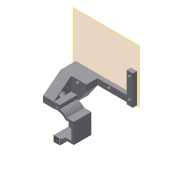
# Autodesk Inventor part: cellSTORM_v5_focusmotormount
Saved by Autodesk Inventor 2019 (Build 230136000, 136)
## iProperties
Created: 2020-05-04
Part Number: cellSTORM_v5_focusmotormount
Material: Generic
Document SubType Name: Modeling
Designer: diederichbenedict
Density: 1 g/cm^3
Appearance: Default
Author: diederichbenedict
Autodesk Inventor part; units mm, degrees
ref_plane "YZ Plane" through (0, 0, 0) normal (1, 0, 0) x (0, 1, 0)
ref_plane "XZ Plane" through (0, 0, 0) normal (0, 1, 0) x (-1, 0, 0)
ref_plane "XY Plane" through (0, 0, 0) normal (0, 0, 1) x (1, 0, 0)
ref_plane "Work Plane1" through (0, 0, 0) normal (0, 0, 1) x (1, 0, 0)
sketch "Sketch1" plane through (0, 0, 0) normal (0, 0, 1) x (1, 0, 0)
  line L0 (-45, 22) -> (22, 22) projected
  line L1 (22, 22) -> (22, -22) projected
  line L2 (22, -22) -> (-45, -22) projected
  line L3 (-45, -28) -> (-45, -22) projected
  line L4 (-30, -28) -> (-45, -28) projected
  line L5 (-30, -28) -> (-28, -30) projected
  line L6 (-28, -30) -> (28, -30) projected
  line L7 (28, -30) -> (30, -28) projected
  line L8 (30, -28) -> (30, 28) projected
  line L9 (30, 28) -> (28, 30) projected
  line L10 (28, 30) -> (-28, 30) projected
  line L11 (-28, 30) -> (-30, 28) projected
  line L12 (-30, 28) -> (-45, 28) projected
  line L13 (-45, 22) -> (-45, 28) projected
  circle A0 centre (25, 25) radius 1.95 projected
  circle A1 centre (25, 0) radius 1.95 projected
  circle A2 centre (0, 25) radius 1.95 projected
  circle A3 centre (-25, -25) radius 1.95 projected
  circle A4 centre (25, -25) radius 1.95 projected
  circle A5 centre (-25, 25) radius 1.95 projected
  circle A6 centre (0, -25) radius 1.95 projected
  line L14 (30, 4.1832) -> (22.5, 4.1832)
  line L15 (22.5, 4.1832) -> (22.5, -32.3594)
  line L16 (22.5, -32.3594) -> (30, -32.3594)
  line L17 (30, -32.3594) -> (30, 4.1832)
  line L18 (22.5, -22.5) -> (-45, -22.5)
  line L19 (-45, -22.5) -> (-45, -30)
  line L20 (-45, -30) -> (22.5, -30)
  line L21 (22.5, -30) -> (22.5, -22.5)
  circle A7 centre (25, 0) radius 2.15
  circle A8 centre (25, -25) radius 2.15
  circle A9 centre (0, -25) radius 2.15
  circle A10 centre (-25, -25) radius 2.15
  point P0 (0, 0)
  dimension "d0" = 0
  dimension "d1" = 0.5
  dimension "d2" = 0.5
  dimension "d3" = 0.2
  dimension "d4" = 0.2
  dimension "d5" = 0.2
  dimension "d6" = 0.2
  constraints: 16 end point, 4 centre point, 4 parallel, 3 point on line, 2 horizontal, 2 perpendicular
  measures "d0" distance between parallel lines of L8 L17
  measures "d1" distance between parallel lines of L1 L15
  measures "d2" distance between parallel lines of L2 L18
  measures "d3" radial gap between concentric circles of A1 A7
  measures "d4" radial gap between concentric circles of A4 A8
  measures "d5" radial gap between concentric circles of A6 A9
  measures "d6" radial gap between concentric circles of A3 A10
extrude "Extrusion1" add sketch "Sketch1" along normal blind 5 contours L18 L15 L6 L5 L4 L3 | L4 L5 L20 L19 | L15 L14 L8 L7 L6 | L6 L7 L17 L16 L15
ref_plane "Work Plane2" through (-32, -78.0277, 40.0715) normal (0, 0, -1) x (0, 1, 0)
sketch "Sketch2" plane through (-32, -78.0277, 40.0715) normal (0, 0, -1) x (0, 1, 0)
  arc A0 (1.8777, 3.5) -> (-2.3223, 3.5) centre (-0.2223, 3.5) ccw projected
  arc A1 (8.5277, 14.4287) -> (3.7223, 7) centre (17.2777, 3.5) ccw projected
  arc A2 (30.8332, 7) -> (26.0277, 14.4287) centre (17.2777, 3.5) ccw projected
  arc A3 (32.6777, 3.5) -> (36.8777, 3.5) centre (34.7777, 3.5) ccw projected
  line L0 (3.7223, 0) -> (-0.2223, 0) projected
  arc A4 (3.2777, 3.5) -> (31.2777, 3.5) centre (17.2777, 3.5) ccw projected
  line L1 (3.2065, 0) -> (-4.2223, 0)
  line L2 (-4.2223, 0) -> (-4.2223, 7.3838)
  line L3 (-4.2223, 7.3838) -> (0.0956, 7.3838)
  line L4 (31.3467, -0.0091) -> (37.7777, -0.0091)
  line L5 (37.7777, -0.0091) -> (38.7777, -0.0091)
  line L6 (38.7777, -0.0091) -> (38.7777, 7.3934)
  line L7 (38.7777, 7.3934) -> (34.4577, 7.3934)
  circle A5 centre (34.7777, 3.5) radius 1.4
  circle A6 centre (-0.2223, 3.5) radius 1.4
  line L8 (8.5277, 22) -> (8.5277, 14.4287)
  line L9 (26.0277, 22) -> (26.0277, 14.4287)
  line L10 (8.0277, 14.6664) -> (5.0277, 14.6664)
  line L11 (5.0277, 14.6664) -> (5.0277, 24.6664)
  line L12 (5.0277, 24.6664) -> (8.0277, 24.6664)
  line L13 (8.0277, 24.6664) -> (8.0277, 14.6664)
  line L14 (26.5277, 14.6664) -> (29.5277, 14.6664)
  line L15 (29.5277, 14.6664) -> (29.5277, 24.6664)
  line L16 (29.5277, 24.6664) -> (26.5277, 24.6664)
  line L17 (26.5277, 24.6664) -> (26.5277, 14.6664)
  line L18 (26.5277, 24.6664) -> (8.0277, 24.6664)
  line L19 (8.0277, 24.6664) -> (8.0277, 21.6664)
  line L20 (8.0277, 21.6664) -> (26.5277, 21.6664)
  line L21 (26.5277, 21.6664) -> (26.5277, 24.6664)
  arc A7 (31.3467, -0.0091) -> (26.5277, 14.6664) centre (17.2777, 3.5) ccw
  arc A8 (8.0277, 14.6664) -> (3.2065, 0) centre (17.2777, 3.5) ccw
  arc A9 (34.4577, 7.3934) -> (29.5277, 16.1589) centre (17.2777, 3.5) ccw
  arc A10 (5.0277, 16.1589) -> (0.0956, 7.3838) centre (17.2777, 3.5) ccw
  point P0 (78.0277, 32)
  dimension "d14" = 2.8
  dimension "d15" = 2.8
  dimension "d16" = 4
  dimension "d17" = 4
  dimension "d33" = 3
  dimension "d34" = 10
  dimension "d35" = 0.5
  dimension "d36" = 3
  dimension "d37" = 3
  dimension "d38" = 10
  constraints: 42 end point, 8 point on circle, 7 perpendicular, 6 centre point, 6 parallel, 5 horizontal, 5 point on line, 4 coincident, 2 vertical, 4 other
  measures "d14" diameter of A5
  measures "d15" diameter of A6
  measures "d16" distance from line of L2 A0.centre
  measures "d17" distance from line of L6 A3.centre
  measures "d33" distance of L11.end L12.end
  measures "d34" distance of L10.end L11.end
  measures "d35" distance between parallel lines of L13 L8
  measures "d36" distance of L16.end L15.end
  measures "d37" distance between parallel lines of L20 L18
  measures "d38" distance between parallel lines of L16 L14
ref_plane "Work Plane3" through (-42.5, -74.75, 21.5715) normal (0, 0, -1) x (0, 1, 0)
extrude "Extrusion2" add sketch "Sketch2" along normal up to surface (18.5 mm away)
sketch "Sketch3" plane through (-24.6066, -39.25, 21.5715) normal (0, 0, -1) x (-1, 0, 0)
  arc A0 (7.4025, -7.431) -> (-7.273, -12.25) centre (3.8934, -21.5) ccw projected
  line L0 (7.4025, 0) -> (7.4025, -7.431) projected
  line L1 (0, 0) -> (7.4025, 0) projected
  line L2 (0, -4.32) -> (0, 0) projected
  arc A1 (0, -4.32) -> (-8.7655, -9.25) centre (3.8934, -21.5) ccw projected
  circle A2 centre (3.8934, -4) radius 1.4 projected
  arc A3 (7.4025, -7.431) -> (-7.273, -12.25) centre (3.8934, -21.5) ccw projected
  line L3 (-17.273, -9.25) -> (-8.7655, -9.25) projected
  line L4 (-14.273, -12.25) -> (-14.273, -30.75) projected
  line L5 (-7.273, -12.25) -> (-14.273, -12.25) projected
  line L6 (-17.273, -33.75) -> (-17.273, -9.25) projected
  line L7 (-8.7655, -33.75) -> (-17.273, -33.75) projected
  arc A4 (-8.7655, -33.75) -> (0.0096, -38.6821) centre (3.8934, -21.5) ccw projected
  line L8 (0.0096, -43) -> (0.0096, -38.6821) projected
  line L9 (7.3934, -43) -> (0.0096, -43) projected
  line L10 (7.3934, -35.5712) -> (7.3934, -43) projected
  arc A5 (-7.273, -30.75) -> (7.3934, -35.5712) centre (3.8934, -21.5) ccw projected
  line L11 (-14.273, -30.75) -> (-7.273, -30.75) projected
  line L12 (7.3934, -35.5712) -> (7.4025, -7.431)
  point P0 (-24.6066, 39.25)
  constraints: 2 end point
extrude "Extrusion3" add sketch "Sketch3" along normal blind 3 contours L12 A5 L11 L4 L5 A0 | A0 L5 L4 L11 A5 L10 L9 L8 A4 L7 L6 L3 A1 L2 L1 L0 | A2
sketch "Sketch4" plane through (0, 0, 5) normal (0, 0, 1) x (1, 0, 0)
  circle A0 centre (25, 0) radius 2.15 projected
  circle A1 centre (25, -25) radius 2.15 projected
  circle A2 centre (-25, -25) radius 2.15 projected
  circle A3 centre (0, -25) radius 2.15 projected
  line L0 (22.5, -22.5) -> (-45, -22.5) projected
  line L1 (-45, -22.5) -> (-45, -30) projected
  line L2 (-45, -30) -> (22.5, -30) projected
  line L3 (22.5, -30) -> (22.5, -32.3594) projected
  line L4 (22.5, -32.3594) -> (30, -32.3594) projected
  line L5 (30, -32.3594) -> (30, 4.1832) projected
  line L6 (30, 4.1832) -> (22.5, 4.1832) projected
  line L7 (22.5, 4.1832) -> (22.5, -22.5) projected
  arc A4 (-25, -47.1946) -> (-32, -47.1946) centre (-28.5, -60.75) ccw projected
  line L8 (-45, -22.5) -> (-45, -30) projected
  arc A5 (-17.3336, -51.5) -> (-32.0091, -46.681) centre (-28.5, -60.75) ccw projected
  line L9 (-45, -22.5) -> (-32.0091, -22.5)
  line L10 (-32.0091, -22.5) -> (-32.0091, -46.681)
  line L11 (-32.0091, -46.681) -> (-45, -46.681)
  line L12 (-45, -46.681) -> (-45, -22.5)
  line L13 (-24.9909, -46.681) -> (-13.3107, -30)
  line L14 (-45, -30) -> (22.5, -30) projected
  line L15 (-24.9909, -46.681) -> (-4.6271, -46.681) construction
  line L16 (-13.3107, -30) -> (-13.3107, -22.5)
  line L17 (22.5, -22.5) -> (-45, -22.5) projected
  point P0 (0, 0)
  point P1 (-32, -74.8212)
  dimension "d20" = 55
  constraints: 14 end point, 2 horizontal, 2 parallel, 2 perpendicular, 2 point on line, 1 equal length, 1 point on circle
  measures "d20" angle of L15 L13
extrude "Extrusion4" add sketch "Sketch4" along normal up to surface (13.5715 mm away) contours L16 L2 L10 L0 | L10 L2 L1 L0 | L13 A5 L10 L2 | L10 L11 L12 L2
sketch "Sketch5" plane through (-45, -30, 0) normal (-1, 0, 0) x (0, 0, 1)
  line L0 (40.0715, -16.681) -> (40.0715, -9.25) projected
  line L1 (40.0715, -9.25) -> (18.5715, -9.25) projected
  line L2 (18.5715, -16.681) -> (18.5715, -9.25) projected
  line L3 (18.5715, -16.681) -> (18.5715, 7.5) projected
  line L4 (40.0715, -16.681) -> (40.0715, -9.25) projected
  line L5 (0, 7.5) -> (18.5715, 7.5) projected
  line L6 (40.0715, -9.25) -> (18.5715, 7.5)
  line L7 (40.0715, -16.681) -> (21.5715, -16.681) projected
  line L8 (21.5715, -16.681) -> (18.5715, -16.681) projected
  point P0 (0, 30)
  constraints: 2 end point
extrude "Extrusion5" add sketch "Sketch5" against normal up to surface (12.9909 mm away)
sketch "Sketch6" plane through (-32.0091, -39.25, 18.5715) normal (1, 0, 0) x (0, 0, -1)
  line L0 (-21.5, 0) -> (0, 0) projected
  line L1 (0, 16.75) -> (0, 0) projected
  line L2 (0, 16.75) -> (-21.5, 0) projected
  circle A0 centre (-10.75, 3.0956) radius 1.4
  point P0 (18.5715, 39.25)
  dimension "d25" = 2.8
  constraints: 1 centre point
  measures "d25" diameter of A0
hole "Hole1" at (-32.0091, -36.1544, 29.3215) direction (-1, 0, 0) diameter 2.8 depth 20 tip angle 118 counterbore diameter 7.5 counterbore depth 4.775
body "Solid1"
